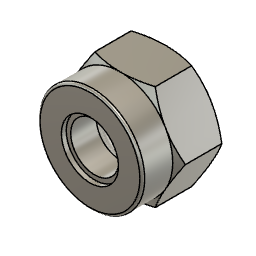
a2587fd3-370a-41ca-846e-29e57ef3b109 (Autodesk Fusion 360 design; units mm, degrees)
description: Hexagon Nut DIN 985 - M3
Autodesk Fusion 360 part; units mm, degrees
sketch "Sketch1" plane through (0, 0, 0) normal (0, 1, 0) x (1, 0, 0)
  line L0 (0, 0) -> (0, -4)
  line L1 (-1.5, 0) -> (-2.75, 0)
  line L2 (-3.1763, -0.2461) -> (-3.1763, -2.1539)
  line L3 (-3.1763, -2.1539) -> (-2.75, -2.4)
  line L4 (-2.75, -2.4) -> (0, -2.4) construction
  line L5 (-3.1763, -0.2461) -> (-2.75, 0)
  line L6 (-2.75, -2.4) -> (-2.75, -4)
  line L7 (-2.75, -4) -> (-1.5, -4)
  line L8 (-1.5, -4) -> (-1.5, -3.7459)
  line L9 (-1.5, -3.7459) -> (-2.4959, -3.7459)
  line L10 (-2.4959, -3.7459) -> (-2.4959, -2.4)
  line L11 (-2.4959, -2.4) -> (-1.5, -2.4)
  line L12 (-1.5, 0) -> (-1.5, -2.4)
  dimension "d127" = 6.3525
  dimension "d140" = 5.5
  dimension "d144" = 30
  dimension "d147" = 30
  dimension "d148" = 2.4
  dimension "d149" = 5.5
  dimension "d150" = 3
  dimension "d151" = 4
  dimension "d152" = 3
  dimension "d153" = 0.2541
  dimension "d154" = 0.2541
  dimension "d155" = 3
  dimension "d187" = 4
  constraint vertical L0
  constraint vertical L2
  constraint coincident L0.start origin
  constraint coincident L0.start L1
  constraint coincident L0 L4.end
  constraint perpendicular L0 L4
  constraint horizontal L1
  constraint perpendicular L4 L6
  constraint perpendicular L6 L7
  constraint perpendicular L7 L8
  constraint perpendicular L8 L9
  constraint coincident L4 L10.end
  constraint perpendicular L4 L10
  constraint coincident L4 L11.end
  measures "d144" angle of L3 L4
  measures "d147" angle of L1 L5
  measures "d148" distance of L1 L3.end
  measures "d151" distance of L1 L6.end
  measures "d153" distance of L7.end L8.end
  measures "d154" distance of L6 L10
  measures "d187" distance of L0.start L0.end
revolve "Revolve4" add sketch "Sketch1" angle 360 about axis through (0, 0, 0) along (0, 0, 1) makes body 1
fillet "Fillet5" radius 0.1271 1 edges at (-2.5639, 0.9944, 4) on bodies 1
sketch "Sketch15" plane through (0, 0, 4) normal (0, 0, 1) x (1, 0, 0)
  circle A0 centre (0, 0) radius 1.5
  circle A1 centre (0, 0) radius 2.6229
  line L0 (0, 0) -> (1.5877, 2.75)
  line L1 (0, 0) -> (-1.5877, 2.75)
  line L2 (-1.5877, 2.75) -> (1.5877, 2.75)
  line L3 (0, 0) -> (0, 5.5) construction
  line L4 (-1.5877, 2.75) -> (1.5877, 2.75)
  line L5 (1.5877, 2.75) -> (1.5877, 3.208)
  line L6 (1.5877, 3.208) -> (-1.5877, 3.208)
  line L7 (-1.5877, 3.208) -> (-1.5877, 2.75)
  dimension "d158" = 60
  dimension "d159" = 60
  dimension "d160" = 2.75
  dimension "d161" = 3.208
  constraint coincident A0.centre A1.centre
  constraint vertical L3
  constraint midpoint L2 L3
  constraint horizontal L4
  constraint vertical L5
  constraint horizontal L6
  constraint vertical L7
  constraint coincident L0.end L2.end
  measures "d158" angle of L0 L1
  measures "d159" angle of L0 L2
  measures "d160" distance of A0.centre L2
  measures "d161" distance of A0.centre L6
extrude "Extrude12" cut sketch "Sketch15" against normal blind 4 contours L2 L4 L5 L6 L7 bodies 1
pattern_circular "C-Pattern3" count 6 over 360 about axis through (0, 0, 1.75) along (0, 0, 1) of "Extrude12"
thread "Thread4" "ISO Metric profile 3.0 M3x0.5 6H" major diameter 3.086 minor diameter 2.529 pitch 0.5 angle 60 resizes the face on face at (-1.4981, 0.0748, 0.8) on bodies 1
sketch "Sketch16" plane through (0, 0, 0) normal (0, 1, 0) x (1, 0, 0)
  line L0 (-2.4959, -3.7459) -> (-2.4959, -2.4)
  line L1 (-2.4959, -2.4) -> (-1.5, -2.4)
  line L2 (-1.5, -3.7459) -> (-2.4959, -3.7459)
  line L3 (1.2645, -2.4) -> (-1.2645, -2.4)
  line L4 (-2.4959, -3.7459) -> (-1.2645, -3.7459)
  line L5 (-1.2645, -3.7459) -> (-1.2645, -2.4)
  line L6 (-1.2645, -2.4) -> (-2.4959, -2.4)
  line L7 (-2.4959, -2.4) -> (-2.4959, -3.7459)
  constraint horizontal L4
  constraint vertical L5
  constraint horizontal L6
  constraint vertical L7
  constraint coincident L3.end L5.end
  constraint coincident L0.start L2.end
revolve "Revolve5" add sketch "Sketch16" angle 360 about axis through (0, 0, 0) along (0, 0, 1) separate body makes body 2
equation "adsk_nheig = 4.00 mm"
equation "adsk_maxdia = 6.3525 mm"
equation "adsk_nomdia = 3.00 mm"
equation "adsk_waflat = 5.50 mm"
equation "d127 = adsk_maxdia"
equation "adsk_baseh = 2.40 mm"
equation "d140 = adsk_waflat"
equation "d144 = adsk_chamang2"
equation "adsk_chamang1 = 30.00 deg"
equation "adsk_chamang2 = 30.00 deg"
equation "d147 = adsk_chamang1"
equation "d148 = adsk_baseh"
equation "d149 = adsk_waflat"
equation "d150 = adsk_nomdia"
equation "d151 = adsk_nheig"
equation "d152 = adsk_nomdia"
equation "d153 = adsk_maxdia * 0.04"
equation "d154 = adsk_maxdia * 0.04"
equation "d155 = adsk_nomdia"
equation "d157 = adsk_maxdia * 0.02"
equation "d160 = adsk_waflat / 2"
equation "d161 = adsk_maxdia / 2 * 1.01"
equation "d162 = -adsk_nheig"
equation "d185 = adsk_nheig"
equation "d187 = adsk_nheig"
